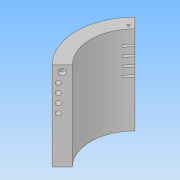
# Autodesk Inventor part: BushingMount
Saved by Autodesk Inventor 2017.3 (Build 213256000, 256)
## iProperties
Created: 2019-06-26
Part Number: BushingMount
Material: Generic
Document SubType Name: Modeling
Designer: Derek Wider
Density: 1 g/cm^3
Appearance: Default
Author: Derek Wider
Autodesk Inventor part; units mm, degrees
ref_plane "YZ Plane" through (0, 0, 0) normal (1, 0, 0) x (0, 1, 0)
ref_plane "XZ Plane" through (0, 0, 0) normal (0, 1, 0) x (-1, 0, 0)
ref_plane "XY Plane" through (0, 0, 0) normal (0, 0, 1) x (1, 0, 0)
sketch "Sketch1" plane through (0, 0, 0) normal (0, 1, 0) x (-1, 0, 0)
  circle A0 centre (0, 0) radius 33.655
  circle A1 centre (0, 0) radius 25.4
  circle A2 centre (0, 0) radius 22.225 construction
  line L0 (17.9605, -17.9605) -> (23.7977, -23.7977)
  line L1 (17.9605, 17.9605) -> (23.7977, 23.7977)
  line L2 (23.7977, 23.7977) -> (0, 23.7977) construction
  line L3 (23.7977, -23.7977) -> (0, -23.7977) construction
  line L4 (0, -23.7977) -> (0, 23.7977) construction
  dimension "d0" = 67.31
  dimension "d1" = 50.8
  dimension "d2" = 44.45
  dimension "d3" = 90
  constraints: 10 end point, 4 point on circle, 3 centre point, 3 coincident, 2 horizontal, 2 line through centre, 1 parallel, 1 vertical, 1 vertical alignment
  measures "d0" diameter of A0
  measures "d1" diameter of A1
  measures "d2" diameter of A2
extrude "Extrusion1" add sketch "Sketch1" along normal blind 50.8 contours A0 L0 A1 L1 picked at (23.2471, 20.152)
sketch "Sketch2" plane through (0, 50.8, 0) normal (0, 1, 0) x (1, 0, 0)
  circle A0 centre (-21.5526, 17.9605) radius 0.762
  line L0 (-17.9605, 17.9605) -> (-23.7977, 23.7977) construction
  arc A1 (-23.7977, 23.7977) -> (-23.7977, -23.7977) centre (0, 0) ccw construction
  line L1 (-23.7977, -23.7977) -> (-17.9605, -17.9605) construction
  arc A2 (-17.9605, 17.9605) -> (-17.9605, -17.9605) centre (0, 0) ccw construction
  line L2 (-17.9605, 17.9605) -> (-29.7034, 6.2177) construction
  arc A3 (-17.9605, 17.9605) -> (-17.9605, -17.9605) centre (0, 0) ccw construction
  dimension "d6" = 2.54
  dimension "d7" = 2.54
  dimension "d8" = 1.524
  constraints: 2 end point, 2 tangent, 1 centre point
  measures "d6" distance from line of L2 A0.centre
  measures "d7" distance from line of L0 A0.centre
  measures "d8" diameter of A0
extrude "Extrusion2" cut sketch "Sketch2" against normal blind 25.4
sketch "Sketch3" plane through (-23.7977, 0, -23.7977) normal (0.7071068, 0, -0.7071068) x (-0.7071068, 0, -0.7071068)
  line L0 (-8.255, 0) -> (0, 0) construction
  line L1 (0, 0) -> (0, 50.8) construction
  line L2 (-8.255, 50.8) -> (0, 50.8) construction
  line L3 (-8.255, 0) -> (-8.255, 50.8) construction
  line L4 (0, 0) -> (0, 50.8) projected
  line L5 (-1.27, 43.18) -> (-10.4633, 43.18)
  line L6 (-10.4633, 43.18) -> (-10.4633, 41.91)
  line L7 (-10.4633, 41.91) -> (-1.27, 41.91)
  line L8 (-1.27, 41.91) -> (-1.27, 43.18)
  point P0 (-33.655, 0)
  dimension "d11" = 41.91
  dimension "d12" = 1.27
  dimension "d18" = 1.27
  constraints: 8 end point, 2 parallel, 1 horizontal, 1 perpendicular
  measures "d11" distance between parallel lines of L7 L0
  measures "d12" distance of L5.end L6.end
  measures "d18" distance between parallel lines of L8 L1
extrude "Extrusion3" cut sketch "Sketch3" against normal blind 5.08
pattern_linear "Rectangular Pattern2" count 4 spacing 5.08 along (0, -1, 0) of "Extrusion3"
sketch "Sketch4" plane through (-17.9605, 0, 17.9605) normal (0.7071068, 0, 0.7071068) x (0.7071068, 0, -0.7071068)
  circle A0 centre (-5.715, 41.91) radius 1.27
  line L0 (-8.255, 0) -> (0, 0) projected
  line L1 (0, 0) -> (0, 50.8) projected
  line L2 (25.4, 0) -> (25.4, 62.631) construction
  circle A1 centre (-5.715, 36.83) radius 1.27
  circle A2 centre (-5.715, 31.75) radius 1.27
  circle A3 centre (-5.715, 26.67) radius 1.27
  dimension "d22" = 2.54
  dimension "d23" = 41.91
  dimension "d24" = 5.715
  dimension "d27" = 5.08
  constraints: 4 centre point, 2 end point, 2 vertical, 6 other
  measures "d22" diameter of A0
  measures "d23" distance from line of A0.centre L0
  measures "d24" distance from line of A0.centre L1
  measures "d27" distance of A0.centre A1.centre
revolve "Revolution1" cut sketch "Sketch4" angle 15 about axis through (0, 0, 0) along (0, -1, 0) contours A0
revolve "Revolution2" cut sketch "Sketch4" angle 25 about axis through (0, 0, 0) along (0, -1, 0) contours A1
revolve "Revolution3" cut sketch "Sketch4" angle 35 about axis through (0, 0, 0) along (0, -1, 0) contours A2
revolve "Revolution4" cut sketch "Sketch4" angle 45 about axis through (0, 0, 0) along (0, -1, 0) contours A3
ref_plane "Work Plane2" through (-29.1461, 0, 16.8275) normal (0.8660254, 0, -0.5) x (0, 1, 0)
ref_plane "Work Plane1" through (0, 0, 0) normal (0.8660254, 0, -0.5) x (0, 1, 0)
sketch "Sketch6" plane through (-29.1461, 0, 16.8275) normal (0.8660254, 0, -0.5) x (0, 1, 0)
  line L0 (40.64, 0) -> (43.18, 0) construction
  line L1 (40.64, 3.175) -> (45.212, 3.175)
  line L2 (45.212, 3.175) -> (45.212, -3.175)
  line L3 (45.212, -3.175) -> (40.64, -3.175)
  line L4 (40.64, -3.175) -> (40.64, 3.175)
  point P0 (0, 0)
  point P1 (45.212, 0)
  dimension "d39" = 4.572
  dimension "d40" = 6.35
  constraints: 8 end point, 2 midpoint, 2 parallel, 1 horizontal, 1 horizontal alignment, 1 perpendicular
  measures "d39" distance of L2.end L3.end
  measures "d40" distance of L1.end L2.end
extrude "Extrusion4" cut sketch "Sketch6" along normal blind 4.064
ref_plane "Work Plane4" through (-31.6254, 0, 11.5107) normal (0.9396926, 0, -0.3420201) x (0, 1, 0)
ref_plane "Work Plane3" through (0, 0, 0) normal (0.9396926, 0, -0.3420201) x (0, 1, 0)
sketch "Sketch7" plane through (-31.6254, 0, 11.5107) normal (0.9396926, 0, -0.3420201) x (0, 1, 0)
  line L0 (35.56, 0) -> (38.1, 0) construction
  line L1 (35.56, -3.175) -> (40.132, -3.175)
  line L2 (40.132, -3.175) -> (40.132, 3.175)
  line L3 (40.132, 3.175) -> (35.56, 3.175)
  line L4 (35.56, 3.175) -> (35.56, -3.175)
  point P0 (0, 0)
  point P1 (40.132, 0)
  dimension "d44" = 6.35
  dimension "d45" = 4.572
  constraints: 8 end point, 2 midpoint, 2 parallel, 1 horizontal, 1 horizontal alignment, 1 perpendicular
  measures "d44" distance between parallel lines of L3 L1
  measures "d45" distance of L1.start L1.end
extrude "Extrusion5" cut sketch "Sketch7" along normal blind 4.064
ref_plane "Work Plane6" through (-33.1437, 0, 5.8441) normal (0.9848078, 0, -0.1736482) x (0, 1, 0)
ref_plane "Work Plane5" through (0, 0, 0) normal (0.9848078, 0, -0.1736482) x (0, 1, 0)
sketch "Sketch8" plane through (-33.1437, 0, 5.8441) normal (0.9848078, 0, -0.1736482) x (0, 1, 0)
  line L0 (30.48, 0) -> (33.02, 0) construction
  line L1 (30.48, 17.8468) -> (30.48, 0) projected
  line L2 (30.48, 3.175) -> (35.052, 3.175)
  line L3 (35.052, 3.175) -> (35.052, -3.175)
  line L4 (35.052, -3.175) -> (30.48, -3.175)
  line L5 (30.48, -3.175) -> (30.48, 3.175)
  point P0 (0, 0)
  point P1 (35.052, 0)
  dimension "d49" = 6.35
  dimension "d50" = 4.572
  constraints: 8 end point, 2 parallel, 1 horizontal, 1 horizontal alignment, 1 midpoint, 1 perpendicular, 1 point on line
  measures "d49" distance between parallel lines of L2 L4
  measures "d50" distance of L3.end L4.end
extrude "Extrusion6" cut sketch "Sketch8" along normal blind 4.064
ref_plane "Work Plane8" through (-33.655, 0, 0) normal (1, 0, 0) x (0, 1, 0)
ref_plane "Work Plane7" through (0, 0, 0) normal (1, 0, 0) x (0, 1, 0)
sketch "Sketch9" plane through (-33.655, 0, 0) normal (1, 0, 0) x (0, 1, 0)
  line L0 (25.4, 0) -> (27.94, 0) projected
  line L1 (25.4, -3.175) -> (29.972, -3.175)
  line L2 (29.972, -3.175) -> (29.972, 3.175)
  line L3 (29.972, 3.175) -> (25.4, 3.175)
  line L4 (25.4, 3.175) -> (25.4, -3.175)
  point P0 (0, 0)
  point P1 (29.972, 0)
  dimension "d54" = 4.572
  dimension "d55" = 6.35
  constraints: 8 end point, 2 midpoint, 2 parallel, 1 horizontal, 1 horizontal alignment, 1 perpendicular
  measures "d54" distance of L1.start L1.end
  measures "d55" distance of L1.end L2.end
extrude "Extrusion7" cut sketch "Sketch9" along normal blind 4.064
sketch "Sketch10" plane through (0, 0, 0) normal (0, -1, 0) x (1, 0, 0)
  circle A0 centre (-30.48, 0) radius 1.27
  point P0 (0, 0)
  dimension "d58" = 2.54
  dimension "d59" = 30.48
  constraints: 1 centre point
  measures "d58" diameter of A0
  measures "d59" distance of A0.centre point (0, 0)
extrude "Extrusion8" cut sketch "Sketch10" against normal blind 12.7
sketch "Sketch11" plane through (-23.7977, 0, -23.7977) normal (0.7071068, 0, -0.7071068) x (-0.7071068, 0, -0.7071068)
  line L0 (-1.27, 26.67) -> (-8.255, 26.67) construction
  line L1 (-8.255, 0) -> (-8.255, 26.67) construction
  line L2 (-8.255, 0) -> (0, 0) construction
  line L3 (0, 0) -> (0, 50.8) construction
  line L4 (-8.255, 50.8) -> (0, 50.8) construction
  line L5 (-8.255, 43.18) -> (-8.255, 50.8) construction
  line L6 (-8.255, 43.18) -> (-1.27, 43.18) construction
  line L7 (-1.27, 43.18) -> (-1.27, 41.91) construction
  line L8 (-1.27, 41.91) -> (-8.255, 41.91) construction
  line L9 (-8.255, 38.1) -> (-8.255, 41.91) construction
  line L10 (-8.255, 38.1) -> (-1.27, 38.1) construction
  line L11 (-1.27, 38.1) -> (-1.27, 36.83) construction
  line L12 (-1.27, 36.83) -> (-8.255, 36.83) construction
  line L13 (-8.255, 33.02) -> (-8.255, 36.83) construction
  line L14 (-8.255, 33.02) -> (-1.27, 33.02) construction
  line L15 (-1.27, 33.02) -> (-1.27, 31.75) construction
  line L16 (-1.27, 31.75) -> (-8.255, 31.75) construction
  line L17 (-8.255, 27.94) -> (-8.255, 31.75) construction
  line L18 (-8.255, 27.94) -> (-1.27, 27.94) construction
  line L19 (-1.27, 27.94) -> (-1.27, 26.67) construction
  circle A0 centre (-4.1275, 47.244) radius 1.778
  point P0 (-33.655, 0)
  dimension "d62" = 3.556
  dimension "d63" = 3.556
  constraints: 1 centre point
  measures "d62" distance from line of A0.centre L4
  measures "d63" diameter of A0
extrude "Extrusion9" cut sketch "Sketch11" against normal through all
sketch "Sketch12" plane through (-17.9605, 0, 17.9605) normal (0.7071068, 0, 0.7071068) x (0.7071068, 0, -0.7071068)
  circle A0 centre (-5.715, 26.67) radius 1.27 construction
  circle A1 centre (-5.715, 31.75) radius 1.27 construction
  circle A2 centre (-5.715, 36.83) radius 1.27 construction
  circle A3 centre (-5.715, 41.91) radius 1.27 construction
  line L0 (-8.255, 0) -> (0, 0) construction
  line L1 (0, 0) -> (0, 50.8) construction
  line L2 (-8.255, 50.8) -> (0, 50.8) construction
  line L3 (-8.255, 0) -> (-8.255, 50.8) construction
  circle A4 centre (-4.1275, 47.244) radius 1.778
  point P0 (25.4, 0)
  dimension "d66" = 3.556
  dimension "d67" = 3.556
  constraints: 1 centre point
  measures "d66" diameter of A4
  measures "d67" distance from line of A4.centre L2
extrude "Extrusion10" cut sketch "Sketch12" against normal through all
ref_plane "Work Plane9" through (-19.7566, 0, 16.1645) normal (0.7071068, 0, 0.7071068) x (0.7071068, 0, -0.7071068)
sketch "Sketch13" plane through (-19.7566, 0, 16.1645) normal (0.7071068, 0, 0.7071068) x (0.7071068, 0, -0.7071068)
  circle A0 centre (-4.1275, 47.244) radius 1.778 construction
  circle A1 centre (-4.1275, 47.244) radius 2.794
  point P0 (25.4, 0)
  dimension "d71" = 5.588
  constraints: 1 centre point, 1 coincident
  measures "d71" diameter of A1
extrude "Extrusion11" cut sketch "Sketch13" against normal through all
ref_plane "Work Plane10" through (-25.5937, 0, -22.0016) normal (0.7071068, 0, -0.7071068) x (-0.7071068, 0, -0.7071068)
sketch "Sketch14" plane through (-25.5937, 0, -22.0016) normal (0.7071068, 0, -0.7071068) x (-0.7071068, 0, -0.7071068)
  circle A0 centre (-4.1275, 47.244) radius 1.778 construction
  circle A1 centre (-4.1275, 47.244) radius 2.794
  point P0 (-33.655, 0)
  dimension "d75" = 5.588
  constraints: 1 centre point, 1 coincident
  measures "d75" diameter of A1
extrude "Extrusion12" cut sketch "Sketch14" against normal through all
body "Solid1"
